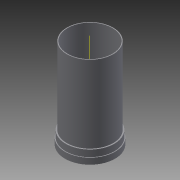
# Autodesk Inventor part: Vacuum Cylinder
Saved by Autodesk Inventor 2015 (Build 190159000, 159)
## iProperties
Created: 2014-07-08
Part Number: Vacuum Cylinder
Material: Generic
Document SubType Name: Modeling
Designer: I Rabey
Density: 1 g/cm^3
Appearance: Default
Author: I Rabey
Autodesk Inventor part; units mm, degrees
sketch "Sketch1" plane through (0, 0, 0) normal (0, 1, 0) x (-1, 0, 0)
  circle A0 centre (0, 0) radius 28.5
  circle A1 centre (0, 0) radius 31.877
  dimension "d0" = 57
  dimension "d1" = 63.754
  constraints: 2 centre point, 2 coincident
  measures "d0" diameter of A0
  measures "d1" diameter of A1
extrude "Extrusion1" add sketch "Sketch1" along normal blind 114.2
ref_plane "Work Plane1" through (0, 7.749, 0) normal (0, 1, 0) x (-1, 0, 0)
sketch "Sketch3" plane through (0, 7.749, 0) normal (0, 1, 0) x (-1, 0, 0)
  circle A0 centre (0, 0) radius 31.877
  circle A1 centre (0, 0) radius 30.988
  dimension "d6" = 61.976
  constraints: 2 centre point, 2 coincident
  measures "d6" diameter of A1
extrude "Extrusion2" cut sketch "Sketch3" along normal blind 200
ref_plane "Work Plane2" through (0, 16.1, 0) normal (0, 1, 0) x (-1, 0, 0)
sketch "Sketch4" plane through (0, 16.1, 0) normal (0, 1, 0) x (-1, 0, 0)
  circle A0 centre (0, 0) radius 29.5
  circle A1 centre (0, 0) radius 27.8909
  circle A2 centre (0, 0) radius 33.2417
  dimension "d10" = 59
  constraints: 3 centre point, 3 coincident
  measures "d10" diameter of A0
extrude "Extrusion3" cut sketch "Sketch4" along normal blind 200 contours A2
ref_plane "Work Plane3" through (0, 113.3, 0) normal (0, 1, 0) x (-1, 0, 0)
body "Solid1"
